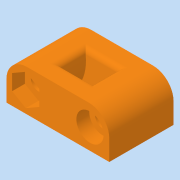
# Autodesk Inventor part: CarriageImproved
Saved by Autodesk Inventor 2017 (Build 210142000, 142)
## iProperties
Created: 2018-04-03
Part Number: CarriageImproved
Material: ABS Plastic
Document SubType Name: Modeling
Designer: Derek Wider
Density: 1.06 g/cm^3
Appearance: Orange
Author: Derek Wider
Autodesk Inventor part; units mm, degrees
ref_plane "YZ Plane" through (0, 0, 0) normal (1, 0, 0) x (0, 1, 0)
ref_plane "XZ Plane" through (0, 0, 0) normal (0, 1, 0) x (-1, 0, 0)
ref_plane "XY Plane" through (0, 0, 0) normal (0, 0, 1) x (1, 0, 0)
sketch "Sketch1" plane through (0, 0, 0) normal (0, 0, 1) x (1, 0, 0)
  circle A0 centre (0, 0) radius 3.3655
  circle A1 centre (0, 0) radius 1.905
  circle A2 centre (-15.875, 0) radius 1.905
  line L0 (-15.875, -3.8861) -> (-19.2405, -1.9431)
  line L1 (-19.2405, -1.9431) -> (-19.2405, 1.9431)
  line L2 (-19.2405, 1.9431) -> (-15.875, 3.8861)
  line L3 (-15.875, 3.8861) -> (-12.5095, 1.9431)
  line L4 (-12.5095, 1.9431) -> (-12.5095, -1.9431)
  line L5 (-12.5095, -1.9431) -> (-15.875, -3.8861)
  line L6 (-20.6375, 5.08) -> (4.7625, 5.08)
  line L7 (4.7625, 5.08) -> (4.7625, -5.08)
  line L8 (4.7625, -5.08) -> (-20.6375, -5.08)
  line L9 (-20.6375, -5.08) -> (-20.6375, 5.08)
  line L10 (3.3655, 0) -> (4.7625, 0) construction
  line L11 (-19.2405, 0) -> (-20.6375, 0) construction
  dimension "d0" = 6.731
  dimension "d1" = 3.81
  dimension "d2" = 3.81
  dimension "d3" = 6.731
  dimension "d4" = 15.875
  dimension "d5" = 10.16
  dimension "d6" = 25.4
  constraints: 24 end point, 3 coincident, 3 horizontal alignment, 3 midpoint, 2 centre point, 2 parallel, 2 perpendicular, 1 collinear, 1 horizontal, 1 vertical, 15 other
  measures "d1" diameter of A1
  measures "d2" diameter of A2
  measures "d3" distance between parallel lines of L4 L1
  measures "d4" distance of A2.centre point (0, 0)
  measures "d5" distance of L6.end L7.end
  measures "d6" distance of L7.end L8.end
extrude "Extrusion1" add sketch "Sketch1" along normal blind 15.875 contours L6 L7 L8 L9
ref_plane "Work Plane1" through (0, 0, 3.175) normal (0, 0, -1) x (-1, 0, 0)
sketch "Sketch2" plane through (0, 0, 3.175) normal (0, 0, -1) x (-1, 0, 0)
  circle A0 centre (0, 0) radius 1.905 projected
  circle A1 centre (0, 0) radius 3.3655 projected
  circle A2 centre (15.875, 0) radius 1.905 projected
  line L0 (19.2405, 1.9431) -> (19.2405, -1.9431) projected
  line L1 (19.2405, -1.9431) -> (15.875, -3.8861) projected
  line L2 (15.875, -3.8861) -> (12.5095, -1.9431) projected
  line L3 (12.5095, -1.9431) -> (12.5095, 1.9431) projected
  line L4 (12.5095, 1.9431) -> (15.875, 3.8861) projected
  line L5 (15.875, 3.8861) -> (19.2405, 1.9431) projected
  circle A3 centre (0, 0) radius 3.3655 projected
  line L6 (20.6375, 5.08) -> (-4.7625, 5.08) projected
  line L7 (-4.7625, 5.08) -> (-4.7625, -5.08) projected
  line L8 (-4.7625, -5.08) -> (20.6375, -5.08) projected
  line L9 (20.6375, -5.08) -> (20.6375, 5.08) projected
extrude "Extrusion2" add sketch "Sketch2" against normal blind 9.525 contours A1 | L0 L1 L2 L3 L4 L5
ref_plane "Work Plane2" through (0, 0, 7.9375) normal (0, 0, -1) x (-1, 0, 0)
sketch "Sketch4" plane through (0, 0, 7.9375) normal (0, 0, -1) x (-1, 0, 0)
  circle A0 centre (0, 0) radius 1.905 construction
  circle A1 centre (15.875, 0) radius 1.905 construction
  line L0 (-4.7625, -5.08) -> (-4.7625, 5.08) construction
  line L1 (-4.7625, 5.08) -> (20.6375, 5.08) construction
  line L2 (20.6375, 5.08) -> (20.6375, -5.08) construction
  line L3 (20.6375, -5.08) -> (-4.7625, -5.08) construction
  line L4 (20.6375, 5.08) -> (-4.7625, 5.08) projected
  line L5 (-4.7625, -5.08) -> (20.6375, -5.08) projected
  arc A2 (12.3825, 5.08) -> (15.0495, -5.08) centre (23.5352, 2.5775) ccw
  line L6 (12.3825, 5.08) -> (4.1275, 5.08)
  line L7 (4.1275, 5.08) -> (4.1275, -5.08)
  line L8 (4.1275, -5.08) -> (15.0495, -5.08)
  dimension "d14" = 11.43
  dimension "d15" = 8.255
  dimension "d16" = 5.588
  dimension "d17" = 8.89
  constraints: 6 end point, 4 point on line, 2 perpendicular, 2 point on circle, 1 centre point
  measures "d14" radius of A2
  measures "d15" distance of L1.end L6.start
  measures "d16" distance of L2.end L8.end
  measures "d17" distance between parallel lines of L0 L7
extrude "Extrusion3" cut sketch "Sketch4" along normal mid plane 6.35
fillet "Fillet3" radius 5.08 2 edges at (-20.6375, 5.08, 7.9375) (4.7625, 5.08, 7.9375)
fillet "Fillet4" radius 1.27 4 edges at (-8.255, 5.08, 4.7625) (-8.255, 5.08, 11.1125) (-4.1275, 5.08, 7.9375) (-12.3825, 5.08, 7.9375)
body "Solid1"
